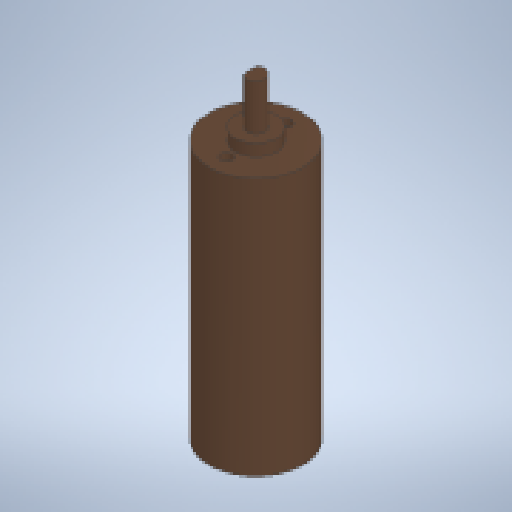
# Autodesk Inventor part: motor2
Saved by Autodesk Inventor 2024 (Build 280153000, 153)
## iProperties
Created: 2022-12-05
Part Number: motor2
Material: Genérico
Document SubType Name: Modeling
Designer: sergi
Density: 1 g/cm^3
Appearance: Valor por defecto
Author: sergi
Autodesk Inventor part; units mm, degrees
ref_plane "YZ Plane" through (0, 0, 0) normal (1, 0, 0) x (0, 1, 0)
ref_plane "XZ Plane" through (0, 0, 0) normal (0, 1, 0) x (-1, 0, 0)
ref_plane "XY Plane" through (0, 0, 0) normal (0, 0, 1) x (1, 0, 0)
sketch "Boceto1" plane through (0, 0, 0) normal (0, 1, 0) x (-1, 0, 0)
  circle A0 centre (0, 0) radius 8
  dimension "d0" = 16
  constraints: 1 centre point, 1 coincident
  measures "d0" diameter of A0
extrude "Extrusión1" add sketch "Boceto1" along normal blind 44
sketch "Boceto2" plane through (0, 44, 0) normal (0, 1, 0) x (1, 0, 0)
  circle A0 centre (0, 0) radius 3.5
  dimension "d3" = 7
  constraints: 1 centre point, 1 coincident
  measures "d3" diameter of A0
extrude "Extrusión2" add sketch "Boceto2" along normal blind 2
sketch "Boceto3" plane through (0, 46, 0) normal (0, 1, 0) x (1, 0, 0)
  arc A0 (-1, -1.118) -> (-1, 1.118) centre (0, 0) ccw
  line L0 (1.5, 0) -> (-1, 0)
  line L1 (-1, 0) -> (-1, 1.118)
  line L2 (-1, 0) -> (-1, -1.118)
  dimension "d6" = 3
  dimension "d7" = 2.5
  constraints: 6 end point, 3 point on circle, 1 centre point, 1 coincident, 1 horizontal, 1 point on line, 1 vertical
  measures "d6" diameter of A0
  measures "d7" distance of L0.start L0.end
extrude "Extrusión3" add sketch "Boceto3" along normal blind 7.8
sketch "Boceto4" plane through (0, 46, 0) normal (0, 1, 0) x (1, 0, 0)
  line L0 (-1, 1.118) -> (-1, -1.118) projected
  circle A0 centre (0, 0) radius 1.5
  constraints: 1 coincident, 3 other
extrude "Extrusión4" add sketch "Boceto4" along normal blind 1.5 contours L0 A0 picked at (-1.1631, -0.0599)
sketch "Boceto5" plane through (0, 44, 0) normal (0, 1, 0) x (1, 0, 0)
  circle A0 centre (0, 0) radius 1.5 projected
  circle A1 centre (0, 0) radius 5
  circle A2 centre (0, 5) radius 1
  circle A3 centre (0, -5) radius 1
  dimension "d12" = 10
  dimension "d13" = 2
  dimension "d14" = 2
  constraints: 3 centre point, 2 point on circle, 1 coincident
  measures "d12" diameter of A1
  measures "d13" diameter of A2
  measures "d14" diameter of A3
hole "Agujero1" at (0, 44, -5) at (0, 44, 5) direction (0, -1, 0) diameter 2 depth 4 tip angle 118
sketch "Boceto6" plane through (0, 44, 0) normal (0, 1, 0) x (1, 0, 0)
  circle A0 centre (0, 5) radius 1 projected
  line L0 (0, 5) -> (0, -5)
  point P0 (0, 0)
  constraints: 2 end point, 1 vertical
